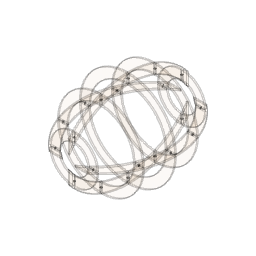
Ljósakróna tilraun v5 (Autodesk Fusion 360 design; units mm, degrees)
Autodesk Fusion 360 part; units mm, degrees
sketch "Sketch2" plane through (0, 0, 0) normal (0, 1, 0) x (1, 0, 0) in component "Hringur minnsti"
  circle A0 centre (0, 0) radius 50
  circle A1 centre (0, 0) radius 30
  dimension "d20" = 100
  dimension "d21" = 60
  constraint coincident A0.centre A1.centre
  measures "d20" diameter of A0
  measures "d21" diameter of A1
extrude "Extrude1" add sketch "Sketch2" along normal blind 3.1 makes body 1 in component "Hringur minnsti"
sketch "Sketch3" plane through (0, 3.1, 0) normal (0, 1, 0) x (-1, 0, 0) in component "Hringur minnsti"
  circle A0 centre (0, 0) radius 30
  circle A1 centre (0, 0) radius 50
  line L0 (-49.976, -1.55) -> (-39.976, -1.55)
  line L1 (-39.976, -1.55) -> (-39.976, 1.55)
  line L2 (-39.976, 1.55) -> (-49.976, 1.55)
  line L3 (0, 0) -> (15.7105, 0)
  dimension "d24" = 10
  dimension "d25" = 3.1
  dimension "d26" = 10
  constraint coincident A1 L0.start
  constraint horizontal L0
  constraint perpendicular L0 L1
  constraint perpendicular L1 L2
  constraint coincident A0.centre A1.centre
  constraint horizontal L3
  constraint symmetric L0 L2 L3
  measures "d24" distance of L0.start L0.end
  measures "d25" distance of L0.end L1.end
  measures "d26" distance of L1.end L2.end
extrude "Extrude2" cut sketch "Sketch3" against normal blind 3.1 contours A1 L0 L1 L2 picked at (-43.3164, 0.1722) bodies 1 in component "Hringur minnsti"
pattern_circular "C-Pattern1" count 4 over 360 about axis through (0, 1.75, 0) along (0, 1, 0) of "Extrude2" in component "Hringur minnsti"
sketch "Sketch1" plane through (0, 0, 0) normal (0, 1, 0) x (1, 0, 0) in component "Hringur miðja"
  circle A0 centre (0, 0) radius 90
  circle A1 centre (0, 0) radius 70
  dimension "d31" = 180
  dimension "d32" = 140
  constraint coincident A0.centre A1.centre
  constraint concentric A0 A1
  measures "d31" diameter of A0
  measures "d32" diameter of A1
extrude "Extrude1'" add sketch "Sketch1" along normal blind 3.1 separate body makes body 2 in component "Hringur miðja"
sketch "Sketch2 (2)" plane through (0, 3.1, 0) normal (0, 1, 0) x (-1, 0, 0) in component "Hringur miðja"
  circle A0 centre (0, 0) radius 70
  circle A1 centre (0, 0) radius 90
  line L0 (-89.9867, -1.55) -> (-79.9867, -1.55)
  line L1 (-79.9867, -1.55) -> (-79.9867, 1.55)
  line L2 (-79.9867, 1.55) -> (-89.9867, 1.55)
  line L3 (0, 0) -> (6.9922, 0)
  dimension "d35" = 10
  dimension "d36" = 3.1
  dimension "d37" = 10
  constraint coincident A1 L0.start
  constraint horizontal L0
  constraint perpendicular L0 L1
  constraint perpendicular L1 L2
  constraint coincident A0.centre A1.centre
  constraint horizontal L3
  constraint symmetric L0 L2 L3
  measures "d35" distance of L0.start L0.end
  measures "d36" distance of L0.end L1.end
  measures "d37" distance of L1.end L2.end
extrude "Extrude2'" cut sketch "Sketch2 (2)" against normal blind 3.1 contours A1 L0 L1 L2 picked at (-83.3239, 0.1722) bodies 2 in component "Hringur miðja"
pattern_circular "C-Pattern1'" count 4 over 360 about axis through (0, 1.75, 0) along (0, 1, 0) of "Extrude2'" in component "Hringur miðja"
sketch "Sketch1 (2)" plane through (0, 0, 0) normal (0, 1, 0) x (1, 0, 0) in component "Hringur stór"
  circle A0 centre (0, 0) radius 100.5
  circle A1 centre (0, 0) radius 80.5
  dimension "d42" = 201
  dimension "d43" = 161
  constraint coincident A0.centre A1.centre
  measures "d42" diameter of A0
  measures "d43" diameter of A1
extrude "Extrude1''" add sketch "Sketch1 (2)" along normal blind 3.1 separate body makes body 3 in component "Hringur stór"
sketch "Sketch2 (3)" plane through (0, 3.1, 0) normal (0, 1, 0) x (-1, 0, 0) in component "Hringur stór"
  circle A0 centre (0, 0) radius 80.5
  circle A1 centre (0, 0) radius 100.5
  line L0 (-100.488, -1.55) -> (-90.488, -1.55)
  line L1 (-90.488, -1.55) -> (-90.488, 1.55)
  line L2 (-90.488, 1.55) -> (-100.488, 1.55)
  line L3 (0, 0) -> (29.4999, 0)
  dimension "d46" = 10
  dimension "d47" = 3.1
  dimension "d48" = 10
  constraint coincident A1 L0.start
  constraint horizontal L0
  constraint perpendicular L0 L1
  constraint perpendicular L1 L2
  constraint coincident A0.centre A1.centre
  constraint horizontal L3
  constraint symmetric L0 L2 L3
  measures "d46" distance of L0.start L0.end
  measures "d47" distance of L0.end L1.end
  measures "d48" distance of L1.end L2.end
extrude "Extrude2''" cut sketch "Sketch2 (3)" against normal blind 3.1 contours A1 L0 L1 L2 picked at (-93.8249, 0.1722) bodies 3 in component "Hringur stór"
pattern_circular "C-Pattern1''" count 4 over 360 about axis through (0, 1.75, 0) along (0, 1, 0) of "Extrude2''" in component "Hringur stór"
sketch "Sketch1 (3)" plane through (0, 0, 0) normal (0, 0, 1) x (1, 0, 0) in component "Bogi"
  arc A0 (0, 250) -> (0, 0) centre (100.5, 125) ccw
  line L0 (0, 250) -> (28, 250)
  line L1 (0, 0) -> (28, 0)
  arc A1 (28, 250) -> (28, 0) centre (110.8997, 125) ccw
  line L2 (0, 170) -> (0, 100)
  dimension "d59" = 250
  dimension "d61" = 28
  dimension "d62" = 28
  dimension "d65" = 100.5
  constraint coincident A0.end L1.start
  constraint horizontal L0
  constraint horizontal L1
  constraint tangent A0 A1
  constraint vertical L2
  measures "d59" distance of A0.end A0.start
  measures "d61" distance of A0.start L0.end
  measures "d62" distance of A0.end L1.end
  measures "d65" distance of A0.centre L2
extrude "Extrude1'''" add sketch "Sketch1 (3)" along normal blind 3.1 separate body makes body 4 in component "Bogi"
sketch "Sketch2 (4)" plane through (0, 0, 3.1) normal (0, 0, 1) x (-1, 0, 0) in component "Bogi"
  arc A0 (0, -250) -> (0, 0) centre (-100.5, -125) ccw
  line L0 (0, 0) -> (-28, 0)
  arc A1 (-28, -250) -> (-28, 0) centre (-110.8997, -125) ccw
  line L1 (-28, -250) -> (0, -250)
  line L2 (-11.021, -236.9) -> (-1.021, -236.9)
  line L3 (-1.021, -236.9) -> (-1.021, -240)
  line L4 (-1.021, -240) -> (-14.6066, -240)
  line L5 (28.624, -180.05) -> (38.624, -180.05)
  line L6 (38.624, -180.05) -> (38.624, -183.15)
  line L7 (38.624, -183.15) -> (27.3607, -183.15)
  line L8 (39.0807, -123.2) -> (49.0807, -123.2)
  line L9 (49.0807, -123.2) -> (49.0807, -126.3)
  line L10 (49.0807, -126.3) -> (39.0859, -126.3)
  line L11 (28.4257, -69.45) -> (38.4257, -69.45)
  line L12 (38.4257, -69.45) -> (38.4257, -66.35)
  line L13 (38.4257, -66.35) -> (27.1493, -66.35)
  line L14 (-11.584, -12.6) -> (-1.584, -12.6)
  line L15 (-1.584, -12.6) -> (-1.584, -9.5)
  line L16 (-1.584, -9.5) -> (-15.2069, -9.5)
  point P0 (-40, -210)
  dimension "d76" = 10
  dimension "d77" = 3.1
  dimension "d80" = 10
  dimension "d81" = 3.1
  dimension "d82" = 10
  dimension "d83" = 3.1
  dimension "d84" = 10
  dimension "d85" = 53.75
  dimension "d86" = 53.75
  dimension "d88" = 3.1
  dimension "d89" = 53.75
  dimension "d90" = 10
  dimension "d91" = 10
  dimension "d92" = 3.1
  dimension "d93" = 53.75
  dimension "d94" = 9.5
  constraint coincident A1 L2.start
  constraint horizontal L2
  constraint perpendicular L2 L3
  constraint coincident A1 L4.end
  constraint perpendicular L3 L4
  constraint coincident A1 L5.start
  constraint horizontal L5
  constraint perpendicular L5 L6
  constraint coincident A1 L7.end
  constraint perpendicular L6 L7
  constraint coincident A1 L8.start
  constraint parallel L5 L8
  constraint perpendicular L8 L9
  constraint coincident A1 L10.end
  constraint perpendicular L9 L10
  constraint coincident A1 L11.start
  constraint horizontal L11
  constraint perpendicular L11 L12
  constraint coincident A1 L13.end
  constraint perpendicular L12 L13
  constraint coincident A1 L14.start
  constraint horizontal L14
  constraint perpendicular L14 L15
  constraint coincident A1 L16.end
  constraint perpendicular L15 L16
  measures "d76" distance of L2.start L2.end
  measures "d77" distance of L2.end L3.end
  measures "d80" distance of L5.start L5.end
  measures "d81" distance of L5.end L6.end
  measures "d82" distance of L8.start L8.end
  measures "d83" distance of L8.end L9.end
  measures "d84" distance of L1 L4
  measures "d85" distance of L2 L7
  measures "d86" distance of L5 L10
  measures "d88" distance of L11.end L12.end
  measures "d89" distance of L8 L11
  measures "d90" distance of L14.start L14.end
  measures "d91" distance of L11.start L11.end
  measures "d92" distance of L14.end L15.end
  measures "d93" distance of L13 L14
  measures "d94" distance of L0 L16
extrude "Extrude4" cut sketch "Sketch2 (4)" against normal blind 3.1 contours A1 L2 L3 L4 | A1 L14 L15 L16 | A1 L5 L6 L7 | A1 L11 L12 L13 | A1 L8 L9 L10 bodies 4 in component "Bogi"
move_body "Move1" bodies 4 to x (1, 0, 0) y (0, 1, 0) z (0, 0, 1) at (-124.7482, 6.1413, 4.0859) in component "Bogi"
move_body "Move1'" bodies 3 to x (1, 0, 0) y (0, 1, 0) z (0, 0, 1) at (-91.4461, -8.1194, 68.5213) in component "Hringur stór"
move_body "Move1''" bodies 2 to x (1, 0, 0) y (0, 1, 0) z (0, 0, 1) at (88.8735, 7.2663, -57.6905) in component "Hringur miðja"
move_body "Move2" bodies 4 to x (1, 0, 0) y (0, 1, 0) z (0, 0, 1) at (-7.6161, 232.5704, 16.5961) in component "Bogi"
sketch "Sketch1 (4)" plane through (0, 0, 0) normal (0, 0, 1) x (1, 0, 0) in component "CAM layout"
  line L0 (308.8492, -210.3693) -> (308.8492, -200.3693)
  line L1 (308.8492, -200.3693) -> (305.7492, -200.3693)
  line L2 (305.7492, -200.3693) -> (305.7492, -210.3693)
  arc A0 (308.8492, -210.3693) -> (397.2858, -121.9326) centre (307.2992, -120.3826) ccw
  arc A1 (217.3125, -121.9326) -> (305.7492, -210.3693) centre (307.2992, -120.3826) ccw
  line L3 (217.3125, -121.9326) -> (227.3125, -121.9326)
  line L4 (227.3125, -121.9326) -> (227.3125, -118.8326)
  line L5 (227.3125, -118.8326) -> (217.3125, -118.8326)
  arc A2 (305.7492, -30.396) -> (217.3125, -118.8326) centre (307.2992, -120.3826) ccw
  line L6 (305.7492, -30.396) -> (305.7492, -40.396)
  line L7 (305.7492, -40.396) -> (308.8492, -40.396)
  line L8 (308.8492, -40.396) -> (308.8492, -30.396)
  arc A3 (397.2858, -118.8326) -> (308.8492, -30.396) centre (307.2992, -120.3826) ccw
  line L9 (397.2858, -118.8326) -> (387.2858, -118.8326)
  line L10 (387.2858, -118.8326) -> (387.2858, -121.9326)
  line L11 (387.2858, -121.9326) -> (397.2858, -121.9326)
  circle A4 centre (307.2992, -120.3826) radius 70
  line L12 (311.7234, -171.9602) -> (311.7234, -161.9602)
  line L13 (311.7234, -161.9602) -> (308.6234, -161.9602)
  line L14 (308.6234, -161.9602) -> (308.6234, -171.9602)
  arc A5 (311.7234, -171.9602) -> (360.1493, -123.5342) centre (310.1734, -121.9842) ccw
  arc A6 (260.1974, -123.5342) -> (308.6234, -171.9602) centre (310.1734, -121.9842) ccw
  line L15 (260.1974, -123.5342) -> (270.1974, -123.5342)
  line L16 (270.1974, -123.5342) -> (270.1974, -120.4342)
  line L17 (270.1974, -120.4342) -> (260.1974, -120.4342)
  arc A7 (308.6234, -72.0082) -> (260.1974, -120.4342) centre (310.1734, -121.9842) ccw
  line L18 (308.6234, -72.0082) -> (308.6234, -82.0082)
  line L19 (308.6234, -82.0082) -> (311.7234, -82.0082)
  line L20 (311.7234, -82.0082) -> (311.7234, -72.0082)
  arc A8 (360.1493, -120.4342) -> (311.7234, -72.0082) centre (310.1734, -121.9842) ccw
  line L21 (360.1493, -120.4342) -> (350.1493, -120.4342)
  line L22 (350.1493, -120.4342) -> (350.1493, -123.5342)
  line L23 (350.1493, -123.5342) -> (360.1493, -123.5342)
  circle A9 centre (310.1734, -121.9842) radius 30
  line L24 (117.0398, -204.7285) -> (117.0398, -194.7285)
  line L25 (117.0398, -194.7285) -> (113.9398, -194.7285)
  line L26 (113.9398, -194.7285) -> (113.9398, -204.7285)
  arc A10 (117.0398, -204.7285) -> (205.4764, -116.2919) centre (115.4898, -114.7419) ccw
  arc A11 (25.5031, -116.2919) -> (113.9398, -204.7285) centre (115.4898, -114.7419) ccw
  line L27 (25.5031, -116.2919) -> (35.5031, -116.2919)
  line L28 (35.5031, -116.2919) -> (35.5031, -113.1919)
  line L29 (35.5031, -113.1919) -> (25.5031, -113.1919)
  arc A12 (113.9398, -24.7552) -> (25.5031, -113.1919) centre (115.4898, -114.7419) ccw
  line L30 (113.9398, -24.7552) -> (113.9398, -34.7552)
  line L31 (113.9398, -34.7552) -> (117.0398, -34.7552)
  line L32 (117.0398, -34.7552) -> (117.0398, -24.7552)
  arc A13 (205.4764, -113.1919) -> (117.0398, -24.7552) centre (115.4898, -114.7419) ccw
  line L33 (205.4764, -113.1919) -> (195.4764, -113.1919)
  line L34 (195.4764, -113.1919) -> (195.4764, -116.2919)
  line L35 (195.4764, -116.2919) -> (205.4764, -116.2919)
  circle A14 centre (115.4898, -114.7419) radius 70
  line L36 (40.8256, -343.6884) -> (30.8256, -343.6884)
  line L37 (30.8256, -346.7884) -> (40.8204, -346.7884)
  line L38 (30.8256, -343.6884) -> (30.8256, -346.7884)
  line L39 (51.2823, -400.5384) -> (41.2823, -400.5384)
  line L40 (41.2823, -403.6384) -> (52.5456, -403.6384)
  line L41 (41.2823, -400.5384) -> (41.2823, -403.6384)
  line L42 (41.4806, -286.8384) -> (41.4806, -289.9384)
  line L43 (52.757, -286.8384) -> (41.4806, -286.8384)
  line L44 (41.4806, -289.9384) -> (51.4806, -289.9384)
  line L45 (90.9273, -457.3884) -> (80.9273, -457.3884)
  line L46 (80.9273, -460.4884) -> (94.5129, -460.4884)
  line L47 (80.9273, -457.3884) -> (80.9273, -460.4884)
  line L48 (81.4903, -229.9884) -> (81.4903, -233.0884)
  line L49 (95.1132, -229.9884) -> (81.4903, -229.9884)
  line L50 (81.4903, -233.0884) -> (91.4903, -233.0884)
  arc A15 (107.9063, -220.4884) -> (95.1132, -229.9884) centre (190.806, -345.4884) ccw
  arc A16 (94.5129, -460.4884) -> (107.9063, -470.4884) centre (190.806, -345.4884) ccw
  arc A17 (91.4903, -233.0884) -> (52.757, -286.8384) centre (190.806, -345.4884) ccw
  arc A18 (52.5456, -403.6384) -> (90.9273, -457.3884) centre (190.806, -345.4884) ccw
  arc A19 (51.4806, -289.9384) -> (40.8256, -343.6884) centre (190.806, -345.4884) ccw
  line L51 (107.9063, -470.4884) -> (79.9063, -470.4884)
  arc A20 (40.8204, -346.7884) -> (51.2823, -400.5384) centre (190.806, -345.4884) ccw
  line L52 (79.9063, -220.4884) -> (107.9063, -220.4884)
  arc A21 (79.9063, -220.4884) -> (79.9063, -470.4884) centre (180.4063, -345.4884) ccw
  line L53 (182.8889, -446.0613) -> (182.8889, -436.0613)
  line L54 (182.8889, -436.0613) -> (179.7889, -436.0613)
  line L55 (179.7889, -436.0613) -> (179.7889, -446.0613)
  arc A22 (182.8889, -446.0613) -> (281.827, -347.1232) centre (181.3389, -345.5732) ccw
  arc A23 (80.8509, -347.1232) -> (179.7889, -446.0613) centre (181.3389, -345.5732) ccw
  line L56 (80.8509, -347.1232) -> (90.8509, -347.1232)
  line L57 (90.8509, -347.1232) -> (90.8509, -344.0232)
  line L58 (90.8509, -344.0232) -> (80.8509, -344.0232)
  arc A24 (179.7889, -245.0852) -> (80.8509, -344.0232) centre (181.3389, -345.5732) ccw
  line L59 (179.7889, -245.0852) -> (179.7889, -255.0852)
  line L60 (179.7889, -255.0852) -> (182.8889, -255.0852)
  line L61 (182.8889, -255.0852) -> (182.8889, -245.0852)
  arc A25 (281.827, -344.0232) -> (182.8889, -245.0852) centre (181.3389, -345.5732) ccw
  line L62 (281.827, -344.0232) -> (271.827, -344.0232)
  line L63 (271.827, -344.0232) -> (271.827, -347.1232)
  line L64 (271.827, -347.1232) -> (281.827, -347.1232)
  circle A26 centre (181.3389, -345.5732) radius 80.5
  line L65 (187.3808, -398.0523) -> (187.3808, -388.0523)
  line L66 (187.3808, -388.0523) -> (184.2808, -388.0523)
  line L67 (184.2808, -388.0523) -> (184.2808, -398.0523)
  arc A27 (187.3808, -398.0523) -> (235.8068, -349.6263) centre (185.8308, -348.0763) ccw
  arc A28 (135.8548, -349.6263) -> (184.2808, -398.0523) centre (185.8308, -348.0763) ccw
  line L68 (135.8548, -349.6263) -> (145.8548, -349.6263)
  line L69 (145.8548, -349.6263) -> (145.8548, -346.5263)
  line L70 (145.8548, -346.5263) -> (135.8548, -346.5263)
  arc A29 (184.2808, -298.1004) -> (135.8548, -346.5263) centre (185.8308, -348.0763) ccw
  line L71 (184.2808, -298.1004) -> (184.2808, -308.1004)
  line L72 (184.2808, -308.1004) -> (187.3808, -308.1004)
  line L73 (187.3808, -308.1004) -> (187.3808, -298.1004)
  arc A30 (235.8068, -346.5263) -> (187.3808, -298.1004) centre (185.8308, -348.0763) ccw
  line L74 (235.8068, -346.5263) -> (225.8068, -346.5263)
  line L75 (225.8068, -346.5263) -> (225.8068, -349.6263)
  line L76 (225.8068, -349.6263) -> (235.8068, -349.6263)
  circle A31 centre (185.8308, -348.0763) radius 30
  line L77 (327.0075, -352.5974) -> (317.0075, -352.5974)
  line L78 (317.0126, -355.6974) -> (327.0075, -355.6974)
  line L79 (327.0075, -355.6974) -> (327.0075, -352.5974)
  line L80 (316.5508, -409.4474) -> (306.5508, -409.4474)
  line L81 (305.2875, -412.5474) -> (316.5508, -412.5474)
  line L82 (316.5508, -412.5474) -> (316.5508, -409.4474)
  line L83 (316.3524, -298.8474) -> (316.3524, -295.7474)
  line L84 (316.3524, -295.7474) -> (305.0761, -295.7474)
  line L85 (306.3524, -298.8474) -> (316.3524, -298.8474)
  line L86 (276.9058, -466.2974) -> (266.9058, -466.2974)
  line L87 (263.3202, -469.3974) -> (276.9058, -469.3974)
  line L88 (276.9058, -469.3974) -> (276.9058, -466.2974)
  line L89 (276.3427, -241.9974) -> (276.3427, -238.8974)
  line L90 (276.3427, -238.8974) -> (262.7199, -238.8974)
  line L91 (266.3427, -241.9974) -> (276.3427, -241.9974)
  arc A32 (317.0075, -352.5974) -> (306.3524, -298.8474) centre (167.0271, -354.3974) ccw
  arc A33 (305.0761, -295.7474) -> (266.3427, -241.9974) centre (167.0271, -354.3974) ccw
  arc A34 (262.7199, -238.8974) -> (249.9268, -229.3974) centre (167.0271, -354.3974) ccw
  line L92 (277.9268, -229.3974) -> (249.9268, -229.3974)
  arc A35 (277.9268, -479.3974) -> (277.9268, -229.3974) centre (177.4268, -354.3974) ccw
  line L93 (277.9268, -479.3974) -> (249.9268, -479.3974)
  arc A36 (249.9268, -479.3974) -> (263.3202, -469.3974) centre (167.0271, -354.3974) ccw
  arc A37 (266.9058, -466.2974) -> (305.2875, -412.5474) centre (167.0271, -354.3974) ccw
  arc A38 (306.5508, -409.4474) -> (317.0126, -355.6974) centre (167.0271, -354.3974) ccw
  line L94 (384.4063, -349.3855) -> (374.4063, -349.3855)
  line L95 (374.4115, -352.4855) -> (384.4063, -352.4855)
  line L96 (384.4063, -352.4855) -> (384.4063, -349.3855)
  line L97 (373.9496, -406.2355) -> (363.9496, -406.2355)
  line L98 (362.6863, -409.3355) -> (373.9496, -409.3355)
  line L99 (373.9496, -409.3355) -> (373.9496, -406.2355)
  line L100 (373.7513, -295.6355) -> (373.7513, -292.5355)
  line L101 (373.7513, -292.5355) -> (362.4749, -292.5355)
  line L102 (363.7513, -295.6355) -> (373.7513, -295.6355)
  line L103 (334.3046, -463.0855) -> (324.3046, -463.0855)
  line L104 (320.719, -466.1855) -> (334.3046, -466.1855)
  line L105 (334.3046, -466.1855) -> (334.3046, -463.0855)
  line L106 (333.7416, -238.7855) -> (333.7416, -235.6855)
  line L107 (333.7416, -235.6855) -> (320.1187, -235.6855)
  line L108 (323.7416, -238.7855) -> (333.7416, -238.7855)
  arc A39 (374.4063, -349.3855) -> (363.7513, -295.6355) centre (224.4259, -351.1855) ccw
  arc A40 (362.4749, -292.5355) -> (323.7416, -238.7855) centre (224.4259, -351.1855) ccw
  arc A41 (320.1187, -235.6855) -> (307.3256, -226.1855) centre (224.4259, -351.1855) ccw
  line L109 (335.3256, -226.1855) -> (307.3256, -226.1855)
  arc A42 (335.3256, -476.1855) -> (335.3256, -226.1855) centre (234.8256, -351.1855) ccw
  line L110 (335.3256, -476.1855) -> (307.3256, -476.1855)
  arc A43 (307.3256, -476.1855) -> (320.719, -466.1855) centre (224.4259, -351.1855) ccw
  arc A44 (324.3046, -463.0855) -> (362.6863, -409.3355) centre (224.4259, -351.1855) ccw
  arc A45 (363.9496, -406.2355) -> (374.4115, -352.4855) centre (224.4259, -351.1855) ccw
  line L111 (436.7612, -351.3342) -> (426.7612, -351.3342)
  line L112 (426.7664, -354.4342) -> (436.7612, -354.4342)
  line L113 (436.7612, -354.4342) -> (436.7612, -351.3342)
  line L114 (426.3045, -408.1842) -> (416.3045, -408.1842)
  line L115 (415.0412, -411.2842) -> (426.3045, -411.2842)
  line L116 (426.3045, -411.2842) -> (426.3045, -408.1842)
  line L117 (426.1062, -297.5842) -> (426.1062, -294.4842)
  line L118 (426.1062, -294.4842) -> (414.8299, -294.4842)
  line L119 (416.1062, -297.5842) -> (426.1062, -297.5842)
  line L120 (386.6595, -465.0342) -> (376.6595, -465.0342)
  line L121 (373.0739, -468.1342) -> (386.6595, -468.1342)
  line L122 (386.6595, -468.1342) -> (386.6595, -465.0342)
  line L123 (386.0965, -240.7342) -> (386.0965, -237.6342)
  line L124 (386.0965, -237.6342) -> (372.4736, -237.6342)
  line L125 (376.0965, -240.7342) -> (386.0965, -240.7342)
  arc A46 (426.7612, -351.3342) -> (416.1062, -297.5842) centre (276.7808, -353.1342) ccw
  arc A47 (414.8299, -294.4842) -> (376.0965, -240.7342) centre (276.7808, -353.1342) ccw
  arc A48 (372.4736, -237.6342) -> (359.6805, -228.1342) centre (276.7808, -353.1342) ccw
  line L126 (387.6805, -228.1342) -> (359.6805, -228.1342)
  arc A49 (387.6805, -478.1342) -> (387.6805, -228.1342) centre (287.1805, -353.1342) ccw
  line L127 (387.6805, -478.1342) -> (359.6805, -478.1342)
  arc A50 (359.6805, -478.1342) -> (373.0739, -468.1342) centre (276.7808, -353.1342) ccw
  arc A51 (376.6595, -465.0342) -> (415.0412, -411.2842) centre (276.7808, -353.1342) ccw
  arc A52 (416.3045, -408.1842) -> (426.7664, -354.4342) centre (276.7808, -353.1342) ccw
component "3D partar og assembly" placed x (1, 0, 0) y (0, 1, 0) z (0, 0, 1) at (0, 0, 0)
component "CAM layout" placed x (1, 0, 0) y (0, 1, 0) z (0, 0, 1) at (0, 0, 0)
component "Hringur minnsti" placed x (0, 0, -1) y (0, 1, 0) z (1, 0, 0) at (-90.8043, 475.6117, 22.795) in component "3D partar og assembly"
component "Hringur miðja" placed x (0, 0, 1) y (0, -1, 0) z (1, 0, 0) at (-33.1137, 315.4279, -66.2758) in component "3D partar og assembly"
component "Hringur stór" placed x (0, 0, 1) y (0, -1, 0) z (1, 0, 0) at (-159.3256, 356.8922, 114.0884) in component "3D partar og assembly"
component "Bogi" placed x (1, 0, 0) y (0, 1, 0) z (0, 0, 1) at (0, 0, 0) in component "3D partar og assembly"
component "Bogi" placed x (0, 0, -1) y (0, 1, 0) z (1, 0, 0) at (-113.0362, 0, -68.5723) in component "3D partar og assembly"
component "Bogi" placed x (-1, 0, 0) y (0, 1, 0) z (0, 0, -1) at (-181.6086, 0, 44.4639) in component "3D partar og assembly"
component "Bogi" placed x (0, 0, 1) y (0, -1, 0) z (1, 0, 0) at (-113.0362, 726.9233, 113.5993) in component "3D partar og assembly"
component "Hringur miðja" placed x (0, 0, 1) y (0, -1, 0) z (1, 0, 0) at (-33.1137, 429.1279, -66.0775) in component "3D partar og assembly"
component "Hringur minnsti" placed x (0, 0, 1) y (0, -1, 0) z (1, 0, 0) at (-90.8043, 251.3117, 22.232) in component "3D partar og assembly"
component "Assembly" placed x (1, 0, 0) y (0, 1, 0) z (0, 0, 1) at (0, 0, 0) in component "3D partar og assembly"
component "Hringur minnsti" placed x (1, 0, 0) y (0, 0, 1) z (0, -1, 0) at (185.8308, -348.0763, -16.5297) in component "CAM layout"
component "Hringur miðja" placed x (1, 0, 0) y (0, 0, 1) z (0, -1, 0) at (26.6163, -172.4324, -23.796) in component "CAM layout"
component "Hringur stór" placed x (1, 0, 0) y (0, 0, 1) z (0, -1, 0) at (272.785, -277.0519, -8.4103) in component "CAM layout"
component "Bogi" placed x (-1, 0, 0) y (0, -1, 0) z (0, 0, 1) at (202.9613, 12.5262, -37.2117) in component "CAM layout"
component "Bogi" placed x (-1, 0, 0) y (0, -1, 0) z (0, 0, 1) at (145.5625, 9.3143, -37.2117) in component "CAM layout"
component "Bogi" placed x (1, 0, 0) y (0, -1, 0) z (0, 0, -1) at (212.2706, 18.2233, 7.1522) in component "CAM layout"
component "Bogi" placed x (-1, 0, 0) y (0, -1, 0) z (0, 0, 1) at (255.3162, 10.5775, -37.2117) in component "CAM layout"
component "Hringur miðja" placed x (1, 0, 0) y (0, 0, 1) z (0, -1, 0) at (218.4257, -178.0732, -23.796) in component "CAM layout"
component "Hringur minnsti" placed x (1, 0, 0) y (0, 0, 1) z (0, -1, 0) at (310.1734, -121.9842, -16.5297) in component "CAM layout"
equation "Hæð = Þvermál1 * 2.5"
equation "Þvermál1 = 100 mm"
equation "Þvermál2 = Þvermál1 * 1.8"
equation "Þvermál3 = Þvermál1 * 2.01"
equation "Þykkt = 3.1 mm"
equation "Breiddhring = Þvermál1 * 0.4"
equation "lfingur = Breiddhring / 4"
equation "dfingur = Þykkt"
equation "nfingur = 4"
equation "d20 = Þvermál1"
equation "d21 = Þvermál1 - Breiddhring"
equation "d22 = Þykkt"
equation "d24 = lfingur"
equation "d25 = dfingur"
equation "d26 = lfingur"
equation "d27 = -Þykkt"
equation "d29 = nfingur"
equation "d31 = Þvermál2"
equation "d32 = Þvermál2 - Breiddhring"
equation "d33 = Þykkt"
equation "d35 = lfingur"
equation "d36 = dfingur"
equation "d37 = lfingur"
equation "d38 = -Þykkt"
equation "d40 = nfingur"
equation "d42 = Þvermál3"
equation "d43 = Þvermál3 - Breiddhring"
equation "d44 = Þykkt"
equation "d46 = lfingur"
equation "d47 = dfingur"
equation "d48 = lfingur"
equation "d49 = -Þykkt"
equation "d51 = nfingur"
equation "Breiddbogi = Breiddhring * 0.7"
equation "d59 = Hæð"
equation "d61 = Breiddbogi"
equation "d62 = Breiddbogi"
equation "d63 = Þykkt"
equation "d65 = Þvermál3 / 2"
equation "nhringir = 5"
equation "bilmillihringja = ( Hæð - 35 mm ) / ( nhringir - 1 )"
equation "hfrtopp = 10 mm"
equation "d76 = lfingur"
equation "d77 = dfingur"
equation "d80 = lfingur"
equation "d81 = dfingur"
equation "d82 = lfingur"
equation "d83 = dfingur"
equation "d84 = hfrtopp"
equation "d85 = bilmillihringja"
equation "d86 = bilmillihringja"
equation "d88 = dfingur"
equation "d89 = bilmillihringja"
equation "d90 = lfingur"
equation "d91 = lfingur"
equation "d92 = dfingur"
equation "d93 = bilmillihringja"
equation "d97 = -Þykkt"
equation "kerf = 0.0118 mm"
equation "half = kerf / 2"
